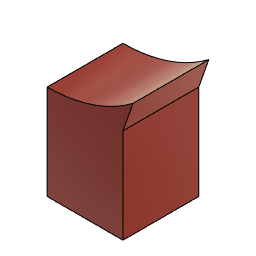
final lamp (Autodesk Fusion 360 archive; units mm, degrees)
design "switch"
Autodesk Fusion 360 part; units mm, degrees
sketch "Sketch1" plane through (0, 0, 0) normal (0, 1, 0) x (1, 0, 0)
  line L0 (0, 0) -> (8, 0)
  line L1 (8, 0) -> (8, -10)
  line L2 (0, -10) -> (0, 0)
  line L3 (8, -10) -> (9.0653, -13.0493)
  arc A0 (9.0653, -13.0493) -> (0, -10) centre (0, -25) ccw
  constraint horizontal L0
  constraint vertical L1
  constraint vertical L2
  constraint coincident L0.start L2.end
extrude "Extrude1" add sketch "Sketch1" along normal blind 8

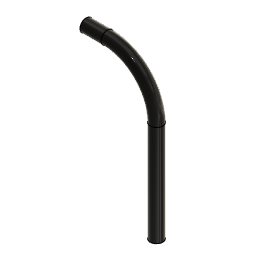
design "rod final"
Autodesk Fusion 360 part; units mm, degrees
sketch "Sketch1" plane through (0, 0, 0) normal (0, 1, 0) x (1, 0, 0)
  line L0 (50, 0) -> (50, -68.58)
  line L1 (-66.42, -185) -> (-116.42, -185)
  arc A0 (-66.42, -185) -> (50, -68.58) centre (-66.42, -68.58) ccw
  constraint vertical L0
ref_plane "WorkPlane1" through (0, 0, 10) normal (0, 0, 1) x (1, 0, 0)
sketch "Sketch2" plane through (0, 0, 0) normal (0, 0, 1) x (1, 0, 0)
  circle A0 centre (50, 0) radius 13
  circle A1 centre (50, 0) radius 15
  constraint concentric A0 A1
sweep "Sweep1" add profiles "Sketch2" path "Sketch1" along L1 A0 L0 section 1
extrude "Extrude1" add 1 faces at (64.2291, -1.3911, 0) along direction (0, 0, -1) blind 170
